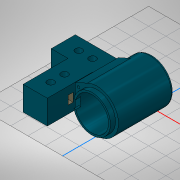
# Autodesk Inventor part: KB33-046-003-001 - Крепление
Saved by Autodesk Inventor 2022 (Build 260153000, 153)
## iProperties
Created: 2021-06-09
Part Number: KB33-046-003-001 - Крепление
Material: ABS Plastic
Document SubType Name: Modeling
Designer: Петров Иван
Density: 1.06 g/cm^3
Appearance: Smooth - Navy
Mass: 109.376 g
Surface Area: 315.588 cm^2
Volume: 103.185 cm^3
Author: Петров Иван
Autodesk Inventor part; units mm, degrees
ref_plane "XZ Plane" through (0, 0, 0) normal (0, 1, 0) x (-1, 0, 0)
ref_plane "XY Plane" through (0, 0, 0) normal (0, 0, 1) x (1, 0, 0)
sketch "Sketch1" plane through (0, 0, 0) normal (0, 0, 1) x (1, 0, 0)
  circle A0 centre (0, 0) radius 19.25
  circle A1 centre (0, 0) radius 25
  dimension "d0" = 38.5
  dimension "d1" = 50
  constraints: 2 centre point, 2 coincident
  measures "d0" diameter of A0
  measures "d1" diameter of A1
extrude "Extrusion1" add sketch "Sketch1" along normal blind 60
sketch "Sketch2" plane through (0, 0, 0) normal (0, 0, -1) x (-1, 0, 0)
  circle A0 centre (0, 0) radius 25
  arc A1 (5.8029, -9.9286) -> (-5.8029, -9.9286) centre (0, 0) ccw
  arc A2 (-5.8029, -9.9286) -> (5.8029, -9.9286) centre (0, -7) ccw
  circle A3 centre (15, 0) radius 1.25
  circle A4 centre (7.5, 12.9904) radius 1.25
  circle A5 centre (-7.5, 12.9904) radius 1.25
  circle A6 centre (-15, 0) radius 1.25
  circle A7 centre (-7.5, -12.9904) radius 1.25
  circle A8 centre (7.5, -12.9904) radius 1.25
  circle A9 centre (0, -7) radius 6
  arc A10 (4.9608, -10.375) -> (-4.9608, -10.375) centre (0, -7) ccw
  spline S0 degree 3 poles (-4.9608, -10.375) (-4.9106, -10.4487) (-4.858, -10.5225) (-4.8027, -10.5964) knots 0 0 0 0 1 1 1 1
  arc A11 (-4.8027, -10.5964) -> (4.8027, -10.5964) centre (0, -7) ccw
  spline S1 degree 3 poles (4.8027, -10.5964) (4.858, -10.5225) (4.9106, -10.4487) (4.9608, -10.375) knots 0 0 0 0 1 1 1 1
  dimension "d4" = 50
  constraints: 12 centre point, 8 point on circle, 7 other
  measures "d4" diameter of A0
extrude "Extrusion2" add sketch "Sketch2" along normal blind 4 contours A0 | A2 A1
sketch "Sketch3" plane through (0, 0, -4) normal (0, 0, -1) x (-1, 0, 0)
  arc A0 (4.9608, -10.375) -> (-4.9608, -10.375) centre (0, -7) ccw projected
  circle A1 centre (0, -7) radius 6.5
  point P0 (0, 0)
  dimension "d7" = 13
  constraints: 1 centre point, 1 coincident
  measures "d7" diameter of A1
extrude "Extrusion3" cut sketch "Sketch3" against normal blind 4
ref_plane "Work Plane1" through (-25, 0, 0) normal (1, 0, 0) x (0, 1, 0)
sketch "Sketch5" plane through (0, 0, 60) normal (0, 0, 1) x (1, 0, 0)
  circle A0 centre (0, 0) radius 25 projected
  line L0 (-19.2094, -16) -> (-25, -16)
  line L1 (-25, -16) -> (-25, 16)
  line L2 (-25, 16) -> (-19.2094, 16)
  circle A1 centre (0, 0) radius 19.25 projected
  line L3 (-19.2094, 16) -> (-19.2094, 1.25)
  line L4 (-19.2094, -1.25) -> (-19.2094, -16)
  dimension "d84" = 32
  constraints: 10 end point, 4 point on circle, 3 parallel, 1 horizontal, 1 perpendicular, 1 tangent
  measures "d84" distance of L0.end L1.end
extrude "Extrusion4" add sketch "Sketch5" against normal blind 50 contours L3 A1 L4 A0 | A0 L1 L2 | L0 L1 A0 picked at (-20.2622, -9.4719)
fillet "Сопряжение13" radius 386.75 2 edges at (-19.2094, -16, 35) (-19.2094, 16, 35)
sketch "Эскиз26" plane through (-25, -16, 60) normal (-1, 0, 0) x (0, 0, 1)
  line L0 (0, 32) -> (0, 0) projected
  line L1 (0, 32) -> (-50, 32) projected
  line L2 (-50, 16) -> (-50, 32) projected
  line L3 (-50, 0) -> (-50, 16) projected
  line L4 (0, 0) -> (-50, 0) projected
  line L5 (-50, 0) -> (-50, 16) projected
  line L6 (0, 35.25) -> (0, -3.25) projected
  line L7 (-22, 2) -> (-50, 2)
  line L8 (-50, 2) -> (-50, 30)
  line L9 (-50, 30) -> (-22, 30)
  line L10 (-22, 30) -> (-22, 2)
  line L11 (-22, 2) -> (-50, 30) construction
  line L12 (-50, 2) -> (-22, 30) construction
  point P0 (-60, 16)
  point P1 (-36, 16)
  dimension "d104" = 28
  dimension "d105" = 28
  constraints: 12 end point, 2 midpoint, 2 parallel, 1 horizontal, 1 perpendicular, 1 point on line
  measures "d104" distance of L8.end L9.end
  measures "d105" distance of L7.end L8.end
extrude "Выдавливание18" add sketch "Эскиз26" along normal blind 50 contours L9 L10 L7 L3 L2
sketch "Эскиз27" plane through (-25, -14, 10) normal (0, -1, 0) x (1, 0, 0)
  line L0 (-50, 0) -> (-50, 28) projected
  line L1 (-50, 14) -> (-0.4658, 14) construction
  line L2 (0, 50) -> (0, 0) projected
  circle A0 centre (-16, 14) radius 4
  circle A1 centre (-32, 14) radius 4
  line L3 (0, 0) -> (-50, 0) projected
  point P0 (25, -10)
  dimension "d112" = 8
  dimension "d113" = 16
  dimension "d114" = 8
  dimension "d115" = 16
  constraints: 2 centre point, 2 end point, 2 point on line, 1 midpoint, 1 parallel
  measures "d112" diameter of A0
  measures "d113" distance from line of L2 A0.centre
  measures "d114" diameter of A1
  measures "d115" distance of A0.centre A1.centre
extrude "Выдавливание19" cut sketch "Эскиз27" against normal through all
sketch "Эскиз28" plane through (0, 0, -4) normal (0, 0, -1) x (-1, 0, 0)
  circle A0 centre (0, -7) radius 6.5 projected
  circle A1 centre (7.5, -12.9904) radius 1.25 projected
  circle A2 centre (-7.5, -12.9904) radius 1.25 projected
  circle A3 centre (-15, 0) radius 1.25 projected
  circle A4 centre (-7.5, 12.9904) radius 1.25 projected
  circle A5 centre (7.5, 12.9904) radius 1.25 projected
  circle A6 centre (15, 0) radius 1.25 projected
  circle A7 centre (0, 0) radius 25 projected
ref_plane "РабПлоскость8" through (0, 0, 55) normal (0, 0, 1) x (1, 0, 0)
sketch "Эскиз30" plane through (-25, -14, 60) normal (0, 0, 1) x (1, 0, 0)
  arc A0 (0, 14) -> (0, 14) centre (25, 14) ccw projected
  circle A1 centre (3.7279, 27.1339) radius 1.5
  dimension "d120" = 3
  constraints: 1 centre point, 1 point on circle
  measures "d120" diameter of A1
extrude "Выдавливание21" cut sketch "Эскиз30" along normal blind 20 and the other way blind 20 contours A1 A0 | A0 A1 picked at (4.1776, 26.9078) picked at (3.2763, 27.3406)
sketch "Эскиз31" plane through (-25, -14, 55) normal (0, 0, 1) x (1, 0, 0)
  circle A0 centre (3.7279, 27.1339) radius 1.5 projected
  line L0 (0.7282, 25.4014) -> (0.7277, 28.8655)
  line L1 (0.7277, 28.8655) -> (3.7274, 30.598)
  line L2 (3.7274, 30.598) -> (6.7277, 28.8664)
  line L3 (6.7277, 28.8664) -> (6.7282, 25.4023)
  line L4 (6.7282, 25.4023) -> (3.7285, 23.6698)
  line L5 (3.7285, 23.6698) -> (0.7282, 25.4014)
  line L6 (6.7277, 28.8664) -> (6.7277, 33.0152)
  arc A1 (0, 30) -> (14.083, 36.4904) centre (-154.8029, 384.4173) ccw projected
  line L7 (3.7285, 23.6698) -> (0, 23.6698)
  line L8 (0, 28) -> (0, 30) projected
  point P0 (25, 14)
  dimension "d125" = 6
  constraints: 16 end point, 1 coincident, 1 perpendicular, 1 point on circle, 1 vertical, 13 other
  measures "d125" distance between parallel lines of L3 L0
extrude "Выдавливание22" cut sketch "Эскиз31" along normal mid plane 4
ref_plane "РабПлоскость7" through (-75, 0, 38) normal (0, -1, 0) x (1, 0, 0)
mirror "Зеркальное отражение1" about plane through (-75, 0, 38) normal (0, -1, 0) of "Выдавливание21", "Выдавливание22"
sketch "Эскиз32" plane through (0, 0, 60) normal (0, 0, 1) x (1, 0, 0)
  circle A0 centre (0, 0) radius 19.25 projected
  circle A1 centre (0, 0) radius 21.5
  line L0 (-20.9105, -5) -> (-18.5893, -5)
  circle A2 centre (0, 0) radius 19.25 projected
  line L1 (-20.9105, 5) -> (-18.5893, 5)
  line L2 (-25, 0) -> (-25, 16) projected
  line L3 (-25, 0) -> (-23.6385, 0)
  dimension "d128" = 43
  dimension "d129" = 5
  constraints: 6 end point, 4 point on circle, 2 horizontal, 1 centre point, 1 coincident, 1 parallel, 1 other
  measures "d128" diameter of A1
  measures "d129" distance between parallel lines of L3 L1
extrude "Выдавливание23" add sketch "Эскиз32" along normal blind 5.75 contours A0 L1 A1 L0 picked at (20.357, 3.2438)
chamfer "Фаска6" distance 2 angle 45 6 edges at (-13.75, 0, -4) (-6.25, 12.9904, -4) (8.75, 12.9904, -4) (-6.25, -12.9904, -4) (8.75, -12.9904, -4) (16.25, 0, -4)
sketch "Эскиз37" plane through (0, 0, 60) normal (0, 0, 1) x (1, 0, 0)
  arc A0 (-10.917, -22.4904) -> (-10.917, 22.4904) centre (0, 0) ccw projected
  arc A1 (-25, 16) -> (-10.917, 22.4904) centre (-179.8029, 370.4173) ccw projected
  line L0 (-25, 16) -> (-25, -16) projected
  arc A2 (-10.917, -22.4904) -> (-25, -16) centre (-179.8029, -370.4173) ccw projected
  line L1 (-18.5893, 5) -> (-20.9105, 5) projected
  arc A3 (-20.9105, -5) -> (-20.9105, 5) centre (0, 0) ccw projected
  line L2 (-20.9105, -5) -> (-18.5893, -5) projected
  arc A4 (-18.5893, 5) -> (-18.5893, -5) centre (0, 0) ccw projected
fillet "Сопряжение25" radius 2.75 1 edges at (25, 0, -4)
sketch "Эскиз38" plane through (-25, -14, 38) normal (0, 0, 1) x (1, 0, 0)
  line L0 (0, 28) -> (-50, 28) projected
  line L1 (-2.5, 0) -> (-30.5, 0)
  line L2 (-30.5, 0) -> (-30.5, 28)
  line L3 (-30.5, 28) -> (-2.5, 28)
  line L4 (-2.5, 28) -> (-2.5, 0)
  line L5 (0, 30) -> (0, -2) projected
  point P0 (25, 14)
  point P1 (-2.5, 28)
  dimension "d155" = 28
  dimension "d166" = 2.5
  constraints: 8 end point, 2 parallel, 1 horizontal, 1 perpendicular, 1 point on line
  measures "d155" distance of L2.end L3.end
  measures "d166" distance between parallel lines of L5 L4
extrude "Выдавливание28" add sketch "Эскиз38" along normal blind 52
sketch "Эскиз39" plane through (-75, 14, 10) normal (0, 1, 0) x (1, 0, 0)
  line L0 (33.5, -79.0412) -> (33.5, -29.507) construction
  circle A0 centre (33.5, -46) radius 4
  circle A1 centre (33.5, -62) radius 4
  line L1 (19.5, -80) -> (47.5, -80) projected
  line L2 (47.5, -80) -> (19.5, -80) projected
  point P0 (75, 10)
  point P1 (25, -10)
  point P2 (33.5, -80)
  point P3 (33.5, -80)
  dimension "d158" = 8
  dimension "d160" = 8
  dimension "d161" = 16
  constraints: 3 point on line, 2 centre point, 2 end point, 2 midpoint
  measures "d158" diameter of A0
  measures "d160" diameter of A1
  measures "d161" distance of A0.centre A1.centre
extrude "Выдавливание29" cut sketch "Эскиз39" against normal blind 50
sketch "Эскиз40" plane through (-55.5, -14, 38) normal (-1, 0, 0) x (0, 0, 1)
  line L0 (22, 19) -> (27.75, 19) projected
  line L1 (22, 9) -> (27.75, 9) projected
  line L2 (22, 9) -> (27.75, 9)
  line L3 (27.75, 9) -> (27.75, 19)
  line L4 (27.75, 19) -> (22, 19)
  line L5 (22, 19) -> (22, 9)
  point P0 (-38, 14)
  point P1 (27.75, 9)
  point P2 (22, 19)
  constraints: 8 end point, 2 parallel, 1 horizontal, 1 perpendicular
extrude "Выдавливание30" cut sketch "Эскиз40" against normal blind 50
sketch "Эскиз41" plane through (0, 0, 10) normal (0, 0, -1) x (-1, 0, 0)
  point P0 (0, 0)
body "Solid1"
